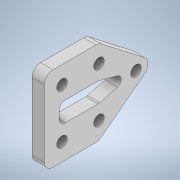
# Autodesk Inventor part: din_motor_connector
Saved by Autodesk Inventor 2021 (Build 250183000, 183)
## iProperties
Created: 2020-11-26
Part Number: din_motor_connector
Material: Generic
Document SubType Name: Modeling
Designer: Mateusz
Density: 1 g/cm^3
Appearance: Default
Author: Mateusz
Autodesk Inventor part; units mm, degrees
ref_plane "YZ Plane" through (0, 0, 0) normal (1, 0, 0) x (0, 1, 0)
ref_plane "XZ Plane" through (0, 0, 0) normal (0, 1, 0) x (-1, 0, 0)
ref_plane "XY Plane" through (0, 0, 0) normal (0, 0, 1) x (1, 0, 0)
sketch "Sketch1" plane through (0, 0, 0) normal (1, 0, 0) x (0, 1, 0)
  circle A0 centre (0, 0) radius 4.25
  circle A1 centre (40, 0) radius 4.25
  circle A2 centre (40, -30) radius 4.25
  circle A3 centre (0, -30) radius 4.25
  circle A4 centre (20, -60) radius 4.25
  line L0 (54.25, 0) -> (54.25, -30)
  line L1 (20, -74.25) -> (54.25, -30)
  line L2 (-14.25, -30) -> (20, -74.25)
  line L3 (-14.25, -30) -> (-14.25, 0)
  line L4 (0, 14.25) -> (54.25, 14.25)
  line L5 (54.25, 14.25) -> (-14.25, 14.25)
  line L6 (-14.25, 14.25) -> (-14.25, 0)
  line L7 (54.25, 14.25) -> (54.25, 0)
  dimension "d6" = 8.5
  dimension "d9" = 8.5
  dimension "d10" = 14.25
  dimension "d11" = 14.25
  dimension "d13" = 14.25
  constraints: 16 end point, 5 centre point, 1 parallel, 1 perpendicular, 1 point on line, 1 vertical
  measures "d6" diameter of A3
  measures "d9" diameter of A4
  measures "d10" distance of A1.centre L0.start
  measures "d11" distance of A4.centre L1.start
  measures "d13" distance of A0.centre L4.start
extrude "Extrusion1" add sketch "Sketch1" along normal blind 10
fillet "Fillet1" radius 7 5 edges at (5, 20, -74.25) (5, 54.25, -30) (5, 54.25, 14.25) (5, -14.25, 14.25) (5, -14.25, -30)
sketch "Sketch2" plane through (10, 0, 0) normal (1, 0, 0) x (0, 0, -1)
  circle A0 centre (0, 40) radius 4.25 projected
  line L0 (0, 28) -> (30, 28)
  line L1 (0, 0) -> (0, 12)
  line L2 (0, 12) -> (30, 12)
  circle A1 centre (60, 20) radius 4.25 projected
  arc A2 (45.061, 16.1433) -> (45.061, 23.8567) centre (44, 20) ccw
  line L3 (30, 28) -> (45.061, 23.8567)
  line L4 (30, 12) -> (45.061, 16.1433)
  line L5 (-14.25, 47.25) -> (-14.25, -7.25) projected
  line L6 (-2.25, 28) -> (0, 28)
  line L7 (-2.25, 28) -> (-2.25, 12)
  line L8 (-2.25, 12) -> (0, 12)
  constraints: 16 end point, 2 point on circle, 2 tangent, 2 vertical, 1 centre point, 1 collinear, 1 perpendicular, 1 point on line
extrude "Extrusion2" cut sketch "Sketch2" against normal up to surface (10 mm away) contours L0 L3 A2 L4 L2 L8 L7 L6
fillet "Fillet2" radius 5 4 edges at (5, 12, -30) (5, 28, -30) (5, 28, 2.25) (5, 12, 2.25)
body "Solid1"
